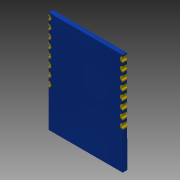
# Autodesk Inventor part: HM-11
Saved by Autodesk Inventor 2013 (Build 170138000, 138)
## iProperties
Created: 2015-07-01
Part Number: HM-11
Material: Ogólny
Document SubType Name: Modeling
Designer: terg
Density: 1 g/cm^3
Author: terg
Autodesk Inventor part; units mm, degrees
ref_plane "YZ Plane" through (0, 0, 0) normal (1, 0, 0) x (0, 1, 0)
ref_plane "XZ Plane" through (0, 0, 0) normal (0, 1, 0) x (-1, 0, 0)
ref_plane "XY Plane" through (0, 0, 0) normal (0, 0, 1) x (1, 0, 0)
sketch "Szkic1" plane through (0, 0, 0) normal (0, 1, 0) x (-1, 0, 0)
  line L0 (0, 0) -> (13.5, 0)
  line L1 (13.5, 0) -> (13.5, -18.5)
  line L2 (13.5, -18.5) -> (0, -18.5)
  line L3 (0, -18.5) -> (0, 0)
  dimension "d0" = 13.5
  dimension "d1" = 18.5
  constraints: 8 end point, 2 parallel, 1 horizontal, 1 perpendicular
  measures "d0" distance of L1.end L2.end
  measures "d1" distance of L0.end L1.end
extrude "Wyciągnięcie proste1" add sketch "Szkic1" along normal blind 0.8
sketch "Szkic2" plane through (0, 0.8, 0) normal (0, 1, 0) x (1, 0, 0)
  line L0 (-13.5, 0) -> (0, 0) projected
  line L1 (-13.5, 18.5) -> (-13.5, 0) projected
  line L2 (-10.5, 8) -> (-4.5, 8)
  line L3 (-4.5, 8) -> (-4.5, 2)
  line L4 (-4.5, 2) -> (-10.5, 2)
  line L5 (-10.5, 2) -> (-10.5, 8)
  dimension "d4" = 6
  dimension "d5" = 6
  dimension "d6" = 2
  dimension "d7" = 3
  constraints: 8 end point, 2 parallel, 1 horizontal, 1 perpendicular
  measures "d4" distance of L3.end L4.end
  measures "d5" distance of L2.end L3.end
  measures "d6" distance between parallel lines of L0 L4
  measures "d7" distance between parallel lines of L1 L5
extrude "Wyciągnięcie proste2" add sketch "Szkic2" along normal blind 0.8
sketch "Szkic3" plane through (0, 0.8, 0) normal (0, 1, 0) x (1, 0, 0)
  line L0 (0, 0) -> (0, 18.5) projected
  line L1 (-13.5, 18.5) -> (0, 18.5)
  line L2 (0, 18.5) -> (0, 13.5)
  line L3 (0, 13.5) -> (-13.5, 13.5)
  line L4 (-13.5, 13.5) -> (-13.5, 18.5)
  dimension "d10" = 5
  constraints: 8 end point, 2 parallel, 1 horizontal, 1 perpendicular, 1 point on line
  measures "d10" distance of L1.end L2.end
extrude "Wyciągnięcie proste3" add sketch "Szkic3" along normal blind 0.01
sketch "Szkic4" plane through (0, 0.81, 0) normal (0, 1, 0) x (1, 0, 0)
  line L0 (0, 18.5) -> (-13.5, 18.5) projected
  line L1 (-13.5, 18.5) -> (-13.5, 13.5) projected
  line L2 (-13.5, 13.5) -> (0, 13.5) projected
  line L3 (-12.7, 13.5) -> (-12.1, 13.5)
  line L4 (-12.1, 13.5) -> (-12.1, 18)
  line L5 (-12.1, 18) -> (-12.7, 18)
  line L6 (-12.7, 18) -> (-12.7, 13.5)
  line L7 (-12.7, 18) -> (-7.7, 18)
  line L8 (-7.7, 18) -> (-7.7, 17.6)
  line L9 (-7.7, 17.6) -> (-12.7, 17.6)
  line L10 (-12.7, 17.6) -> (-12.7, 18)
  line L11 (-10.6, 18) -> (-10.2, 18)
  line L12 (-10.2, 18) -> (-10.2, 13.5)
  line L13 (-10.2, 13.5) -> (-10.6, 13.5)
  line L14 (-10.6, 13.5) -> (-10.6, 18)
  line L15 (-7.7, 18) -> (-8.1, 18)
  line L16 (-8.1, 18) -> (-8.1, 14.5)
  line L17 (-8.1, 14.5) -> (-7.7, 14.5)
  line L18 (-7.7, 14.5) -> (-7.7, 18)
  line L19 (-8.1, 14.5) -> (-6.3, 14.5)
  line L20 (-6.3, 14.5) -> (-6.3, 14.9)
  line L21 (-6.3, 14.9) -> (-8.1, 14.9)
  line L22 (-8.1, 14.9) -> (-8.1, 14.5)
  line L23 (-6.3, 14.5) -> (-5.9, 14.5)
  line L24 (-5.9, 14.5) -> (-5.9, 18)
  line L25 (-5.9, 18) -> (-6.3, 18)
  line L26 (-6.3, 18) -> (-6.3, 14.5)
  line L27 (-6.3, 18) -> (-4.8, 18)
  line L28 (-4.8, 18) -> (-4.8, 17.6)
  line L29 (-4.8, 17.6) -> (-6.3, 17.6)
  line L30 (-6.3, 17.6) -> (-6.3, 18)
  line L31 (-4.8, 18) -> (-4.4, 18)
  line L32 (-4.4, 18) -> (-4.4, 14.5)
  line L33 (-4.4, 14.5) -> (-4.8, 14.5)
  line L34 (-4.8, 14.5) -> (-4.8, 18)
  line L35 (-4.4, 14.5) -> (-3, 14.5)
  line L36 (-3, 14.5) -> (-3, 14.9)
  line L37 (-3, 14.9) -> (-4.4, 14.9)
  line L38 (-4.4, 14.9) -> (-4.4, 14.5)
  line L39 (-3, 14.5) -> (-2.6, 14.5)
  line L40 (-2.6, 14.5) -> (-2.6, 18)
  line L41 (-2.6, 18) -> (-3, 18)
  line L42 (-3, 18) -> (-3, 14.5)
  line L43 (-2.6, 18) -> (-1.2, 18)
  line L44 (-1.2, 18) -> (-1.2, 17.6)
  line L45 (-1.2, 17.6) -> (-2.6, 17.6)
  line L46 (-2.6, 17.6) -> (-2.6, 18)
  line L47 (-1.2, 18) -> (-0.8, 18)
  line L48 (-0.8, 18) -> (-0.8, 14.5)
  line L49 (-0.8, 14.5) -> (-1.2, 14.5)
  line L50 (-1.2, 14.5) -> (-1.2, 18)
  line L51 (0, 13.5) -> (0, 18.5) projected
  point P0 (0, 0)
  dimension "d13" = 0.6
  dimension "d14" = 4.5
  dimension "d15" = 0.5
  dimension "d16" = 0.8
  dimension "d17" = 5
  dimension "d18" = 0.4
  dimension "d19" = 0.4
  dimension "d20" = 1.5
  dimension "d21" = 0.4
  dimension "d22" = 3.5
  dimension "d23" = 1.8
  dimension "d24" = 0.4
  dimension "d25" = 0.4
  dimension "d26" = 3.5
  dimension "d27" = 1.5
  dimension "d28" = 0.4
  dimension "d29" = 0.4
  dimension "d30" = 3.5
  dimension "d31" = 1.4
  dimension "d32" = 0.4
  dimension "d33" = 0.4
  dimension "d34" = 3.5
  dimension "d35" = 1.4
  dimension "d36" = 0.4
  dimension "d37" = 0.4
  dimension "d38" = 3.5
  dimension "d103" = 0.8
  constraints: 96 end point, 24 parallel, 12 horizontal, 12 perpendicular, 2 point on line
  measures "d13" distance of L5.end L4.end
  measures "d14" distance of L4.end L3.end
  measures "d15" distance between parallel lines of L0 L5
  measures "d16" distance between parallel lines of L1 L6
  measures "d17" distance of L8.end L9.end
  measures "d18" distance of L7.end L8.end
  measures "d19" distance of L12.end L13.end
  measures "d20" distance between parallel lines of L4 L14
  measures "d21" distance of L17.end L16.end
  measures "d22" distance of L16.end L15.end
  measures "d23" distance of L21.end L20.end
  measures "d24" distance of L20.end L19.end
  measures "d25" distance of L25.end L24.end
  measures "d26" distance of L24.end L23.end
  measures "d27" distance of L28.end L29.end
  measures "d28" distance of L27.end L28.end
  measures "d29" distance of L32.end L33.end
  measures "d30" distance of L31.end L32.end
  measures "d31" distance of L37.end L36.end
  measures "d32" distance of L35.end L36.end
  measures "d33" distance of L41.end L40.end
  measures "d34" distance of L40.end L39.end
  measures "d35" distance of L44.end L45.end
  measures "d36" distance of L43.end L44.end
  measures "d37" distance of L48.end L49.end
  measures "d38" distance of L47.end L48.end
  measures "d103" distance between parallel lines of L51 L48
extrude "Wyciągnięcie proste4" add sketch "Szkic4" along normal blind 0.01 contours L2 L14 L9 L12 | L6 L9 L4 L2 | L12 L7 L16 L9 | L9 L14 L7 L12 | L6 L5 L4 L9 | L9 L4 L7 L14 | L16 L7 L8 L9 | L9 L18 L21 L16 | L21 L18 L17 L16 | L21 L20 L19 L18 | L26 L29 L24 L23 L20 | L26 L25 L24 L29 | L24 L27 L28 L29 | L28 L31 L32 L33 L34 | L32 L37 L36 L35 | L36 L42 L41 L40 L39 | L40 L43 L44 L45 | L44 L47 L48 L49 L50
sketch "Szkic5" plane through (0, 0.8, 0) normal (0, 1, 0) x (1, 0, 0)
  line L0 (-13.5, 13.5) -> (-13.5, 0) projected
  line L1 (0, 0) -> (0, 13.5) projected
  line L2 (-10.5, 2) -> (-10.5, 8) projected
  line L3 (-10.5, 8) -> (-4.5, 8) projected
  line L4 (-2.8, 11) -> (-1.2, 11)
  line L5 (-1, 10.8) -> (-1, 8.2)
  line L6 (-1.2, 8) -> (-2.8, 8)
  line L7 (-3, 8.2) -> (-3, 10.8)
  line L8 (-12.3, 8.5) -> (-11.7, 8.5)
  line L9 (-11.5, 8.3) -> (-11.5, 5.7)
  line L10 (-11.7, 5.5) -> (-12.3, 5.5)
  line L11 (-12.5, 5.7) -> (-12.5, 8.3)
  arc A0 (-12.3, 8.5) -> (-12.5, 8.3) centre (-12.3, 8.3) ccw
  arc A1 (-11.5, 8.3) -> (-11.7, 8.5) centre (-11.7, 8.3) ccw
  arc A2 (-11.7, 5.5) -> (-11.5, 5.7) centre (-11.7, 5.7) ccw
  arc A3 (-12.5, 5.7) -> (-12.3, 5.5) centre (-12.3, 5.7) ccw
  arc A4 (-3, 8.2) -> (-2.8, 8) centre (-2.8, 8.2) ccw
  arc A5 (-2.8, 11) -> (-3, 10.8) centre (-2.8, 10.8) ccw
  arc A6 (-1, 10.8) -> (-1.2, 11) centre (-1.2, 10.8) ccw
  arc A7 (-1.2, 8) -> (-1, 8.2) centre (-1.2, 8.2) ccw
  point P0 (-3, 11)
  point P1 (-1, 8)
  point P2 (-1, 11)
  point P3 (-3, 8)
  point P4 (-12.5, 8.5)
  point P5 (-11.5, 5.5)
  point P6 (-11.5, 8.5)
  point P7 (-12.5, 5.5)
  dimension "d41" = 2
  dimension "d42" = 3
  dimension "d43" = 1
  dimension "d44" = 3
  dimension "d45" = 1
  dimension "d46" = 1
  dimension "d47" = 1
  dimension "d48" = 0
  dimension "d49" = 0.5
  dimension "d50" = 2.5
  dimension "d53" = 0.2
  constraints: 16 end point, 16 point on circle, 16 point on line, 16 tangent, 8 centre point, 7 equal radius, 4 parallel, 2 horizontal, 2 perpendicular
  measures "d41" distance of point (-1, 8) point (-3, 8)
  measures "d42" distance of point (-1, 11) point (-1, 8)
  measures "d43" distance of point (-11.5, 5.5) point (-12.5, 5.5)
  measures "d44" distance of point (-11.5, 8.5) point (-11.5, 5.5)
  measures "d45" distance between parallel lines of L2 L9
  measures "d46" distance between parallel lines of L0 L11
  measures "d47" distance between parallel lines of L1 L5
  measures "d48" distance between parallel lines of L3 L6
  measures "d49" distance between parallel lines of L8 L3
  measures "d50" distance between parallel lines of L3 L10
  measures "d53" radius of A0
extrude "Wyciągnięcie proste5" add sketch "Szkic5" along normal blind 0.6
chamfer "Faza1" distance 0.2 angle 45 16 edges at (-3, 1.4, -9.5) (-2.9414, 1.4, -8.0586) (-2, 1.4, -8) (-1.0586, 1.4, -8.0586) (-1, 1.4, -9.5) (-1.0586, 1.4, -10.9414) (-2, 1.4, -11) (-2.9414, 1.4, -10.9414) (-11.5, 1.4, -7) (-11.5586, 1.4, -8.4414) (-12, 1.4, -8.5) (-12.4414, 1.4, -8.4414) (-12.5, 1.4, -7) (-12.4414, 1.4, -5.5586) (-12, 1.4, -5.5) (-11.5586, 1.4, -5.5586)
sketch "Szkic6" plane through (0, 0.8, 0) normal (0, 1, 0) x (1, 0, 0)
  line L0 (-13.5, 0) -> (0, 0) projected
  line L1 (0, 0) -> (0, 13.5) projected
  point P0 (0, 0.75)
  point P1 (0, 2.25)
  point P2 (0, 3.75)
  point P3 (0, 5.25)
  point P4 (0, 6.75)
  point P5 (0, 8.25)
  point P6 (0, 9.75)
  point P7 (0, 11.25)
  point P8 (-13.5, 0.75)
  point P9 (-13.5, 2.25)
  point P10 (-13.5, 3.75)
  point P11 (-13.5, 5.25)
  point P12 (-13.5, 6.75)
  point P13 (-13.5, 8.25)
  point P14 (-13.5, 9.75)
  point P15 (-13.5, 11.25)
  dimension "d59" = 1.5
  dimension "d64" = 0.75
  dimension "d67" = 13.5
  constraints: 1 horizontal, 1 point on line, 1 vertical, 16 other
  measures "d59" distance of point (0, 0.75) point (0, 2.25)
  measures "d64" distance from line of L0 point (0, 0.75)
  measures "d67" distance of L0.end point (-13.5, 0)
hole "Otwór1" at (0, 0.8, -0.75) at (0, 0.8, -2.25) at (0, 0.8, -3.75) at (0, 0.8, -5.25) at (0, 0.8, -6.75) at (0, 0.8, -8.25) at (0, 0.8, -9.75) at (0, 0.8, -11.25) at (-13.5, 0.8, -11.25) at (-13.5, 0.8, -9.75) at (-13.5, 0.8, -8.25) at (-13.5, 0.8, -6.75) at (-13.5, 0.8, -5.25) at (-13.5, 0.8, -3.75) at (-13.5, 0.8, -2.25) at (-13.5, 0.8, -0.75) direction (0, -1, 0) diameter 0.5 depth 8
sketch "Szkic7" plane through (0, 0.8, 0) normal (0, 1, 0) x (1, 0, 0)
  line L0 (-13.5, 2) -> (-13.5, 1) projected
  arc A0 (-13.5, 0.5) -> (-13.5, 1) centre (-13.5, 0.75) ccw projected
  line L1 (-13.5, 0.5) -> (-13.5, 0) projected
  line L2 (0, 0) -> (0, 0.5) projected
  arc A1 (0, 1) -> (0, 0.5) centre (0, 0.75) ccw projected
  line L3 (0, 1) -> (0, 2) projected
  line L4 (0, 2.5) -> (0, 3.5) projected
  line L5 (-13.5, 8) -> (-13.5, 7) projected
  line L6 (-13.5, 3.5) -> (-13.5, 2.5) projected
  arc A2 (0.01, 1.2499) -> (0.01, 0.2501) centre (0, 0.75) ccw
  arc A3 (0.01, 0.9998) -> (0.01, 0.5002) centre (0, 0.75) ccw
  line L7 (0.01, 0.9998) -> (0.01, 1.2499)
  line L8 (0.01, 0.5002) -> (0.01, 0.25)
  arc A4 (0.01, 2.7499) -> (0.01, 1.7501) centre (0, 2.25) ccw
  arc A5 (0.01, 2.4998) -> (0.01, 2.0002) centre (0, 2.25) ccw
  line L9 (0.01, 2.4998) -> (0.01, 2.7499)
  line L10 (0.01, 2.0002) -> (0.01, 1.75)
  arc A6 (0.01, 4.2499) -> (0.01, 3.2501) centre (0, 3.75) ccw
  arc A7 (0.01, 3.9998) -> (0.01, 3.5002) centre (0, 3.75) ccw
  line L11 (0.01, 3.9998) -> (0.01, 4.2499)
  line L12 (0.01, 3.5002) -> (0.01, 3.25)
  arc A8 (0.01, 5.7499) -> (0.01, 4.7501) centre (0, 5.25) ccw
  arc A9 (0.01, 5.4998) -> (0.01, 5.0002) centre (0, 5.25) ccw
  line L13 (0.01, 5.4998) -> (0.01, 5.7499)
  line L14 (0.01, 5.0002) -> (0.01, 4.75)
  arc A10 (0.01, 7.2499) -> (0.01, 6.2501) centre (0, 6.75) ccw
  arc A11 (0.01, 6.9998) -> (0.01, 6.5002) centre (0, 6.75) ccw
  line L15 (0.01, 6.9998) -> (0.01, 7.2499)
  line L16 (0.01, 6.5002) -> (0.01, 6.25)
  arc A12 (0.01, 8.7499) -> (0.01, 7.7501) centre (0, 8.25) ccw
  arc A13 (0.01, 8.4998) -> (0.01, 8.0002) centre (0, 8.25) ccw
  line L17 (0.01, 8.4998) -> (0.01, 8.7499)
  line L18 (0.01, 8.0002) -> (0.01, 7.75)
  arc A14 (0.01, 10.2499) -> (0.01, 9.2501) centre (0, 9.75) ccw
  arc A15 (0.01, 9.9998) -> (0.01, 9.5002) centre (0, 9.75) ccw
  line L19 (0.01, 9.9998) -> (0.01, 10.2499)
  line L20 (0.01, 9.5002) -> (0.01, 9.25)
  arc A16 (0.01, 11.7499) -> (0.01, 10.7501) centre (0, 11.25) ccw
  arc A17 (0.01, 11.4998) -> (0.01, 11.0002) centre (0, 11.25) ccw
  line L21 (0.01, 11.4998) -> (0.01, 11.7499)
  line L22 (0.01, 11.0002) -> (0.01, 10.75)
  arc A18 (-13.51, 0.2501) -> (-13.51, 1.2499) centre (-13.5, 0.75) ccw
  arc A19 (-13.51, 0.5002) -> (-13.51, 0.9998) centre (-13.5, 0.75) ccw
  line L23 (-13.51, 1.2499) -> (-13.51, 0.9998)
  line L24 (-13.51, 0.5002) -> (-13.51, 0.2501)
  arc A20 (-13.51, 1.7501) -> (-13.51, 2.7499) centre (-13.5, 2.25) ccw
  arc A21 (-13.51, 2.0002) -> (-13.51, 2.4998) centre (-13.5, 2.25) ccw
  line L25 (-13.51, 2.7499) -> (-13.51, 2.4998)
  line L26 (-13.51, 2.0002) -> (-13.51, 1.7501)
  arc A22 (-13.51, 3.2501) -> (-13.51, 4.2499) centre (-13.5, 3.75) ccw
  arc A23 (-13.51, 3.5002) -> (-13.51, 3.9998) centre (-13.5, 3.75) ccw
  line L27 (-13.51, 4.2499) -> (-13.51, 3.9998)
  line L28 (-13.51, 3.5002) -> (-13.51, 3.2501)
  arc A24 (-13.51, 4.7501) -> (-13.51, 5.7499) centre (-13.5, 5.25) ccw
  arc A25 (-13.51, 5.0002) -> (-13.51, 5.4998) centre (-13.5, 5.25) ccw
  line L29 (-13.51, 5.7499) -> (-13.51, 5.4998)
  line L30 (-13.51, 5.0002) -> (-13.51, 4.7501)
  arc A26 (-13.51, 6.2501) -> (-13.51, 7.2499) centre (-13.5, 6.75) ccw
  arc A27 (-13.51, 6.5002) -> (-13.51, 6.9998) centre (-13.5, 6.75) ccw
  line L31 (-13.51, 7.2499) -> (-13.51, 6.9998)
  line L32 (-13.51, 6.5002) -> (-13.51, 6.2501)
  arc A28 (-13.51, 7.7501) -> (-13.51, 8.7499) centre (-13.5, 8.25) ccw
  arc A29 (-13.51, 8.0002) -> (-13.51, 8.4998) centre (-13.5, 8.25) ccw
  line L33 (-13.51, 8.7499) -> (-13.51, 8.4998)
  line L34 (-13.51, 8.0002) -> (-13.51, 7.7501)
  arc A30 (-13.51, 9.2501) -> (-13.51, 10.2499) centre (-13.5, 9.75) ccw
  arc A31 (-13.51, 9.5002) -> (-13.51, 9.9998) centre (-13.5, 9.75) ccw
  line L35 (-13.51, 10.2499) -> (-13.51, 9.9998)
  line L36 (-13.51, 9.5002) -> (-13.51, 9.2501)
  arc A32 (-13.51, 10.7501) -> (-13.51, 11.7499) centre (-13.5, 11.25) ccw
  arc A33 (-13.51, 11.0002) -> (-13.51, 11.4998) centre (-13.5, 11.25) ccw
  line L37 (-13.51, 11.7499) -> (-13.51, 11.4998)
  line L38 (-13.51, 11.0002) -> (-13.51, 10.7501)
  point P0 (0, 1.5)
  point P1 (0, 2.5)
  point P2 (0, 3)
  point P3 (0, 4)
  point P4 (0, 4.5)
  point P5 (0, 5)
  point P6 (0, 5.5)
  point P7 (0, 6)
  point P8 (0, 6.5)
  point P9 (0, 7)
  point P10 (0, 7.5)
  point P11 (0, 8)
  point P12 (0, 8.5)
  point P13 (0, 9)
  point P14 (0, 9.5)
  point P15 (0, 10)
  point P16 (0, 10.5)
  point P17 (0, 11)
  point P18 (0, 11.5)
  point P19 (-13.5, 2.5)
  point P20 (-13.5, 1.5)
  point P21 (-13.5, 4)
  point P22 (-13.5, 3)
  point P23 (-13.5, 5.5)
  point P24 (-13.5, 5)
  point P25 (-13.5, 4.5)
  point P26 (-13.5, 7)
  point P27 (-13.5, 6.5)
  point P28 (-13.5, 6)
  point P29 (-13.5, 8.5)
  point P30 (-13.5, 7.5)
  point P31 (-13.5, 10)
  point P32 (-13.5, 9.5)
  point P33 (-13.5, 9)
  point P34 (-13.5, 11.5)
  point P35 (-13.5, 11)
  point P36 (-13.5, 10.5)
  dimension "d79" = 1
  dimension "d80" = 0.01
  dimension "d81" = 0.01
  dimension "d84" = 1.5
  dimension "d89" = 1
  dimension "d90" = 0.01
  dimension "d91" = 0.01
  dimension "d94" = 1.5
  constraints: 80 point on circle, 64 end point, 32 centre point, 32 coincident, 8 point on line, 2 collinear, 2 parallel, 2 vertical, 203 other
  measures "d79" diameter of A2
  measures "d80" distance between parallel lines of L3 L7
  measures "d81" distance between parallel lines of L8 L2
  measures "d84" distance of L3.start point (0, 2.5)
  measures "d89" diameter of A18
  measures "d90" distance between parallel lines of L23 L0
  measures "d91" distance between parallel lines of L1 L24
  measures "d94" distance of L1.end point (-13.5, 1.5)
extrude "Wyciągnięcie proste6" add sketch "Szkic7" along normal blind 0.01 and the other way blind 0.81
equation "\"d16\" = d103"
equation "\"d45\" = d46"
